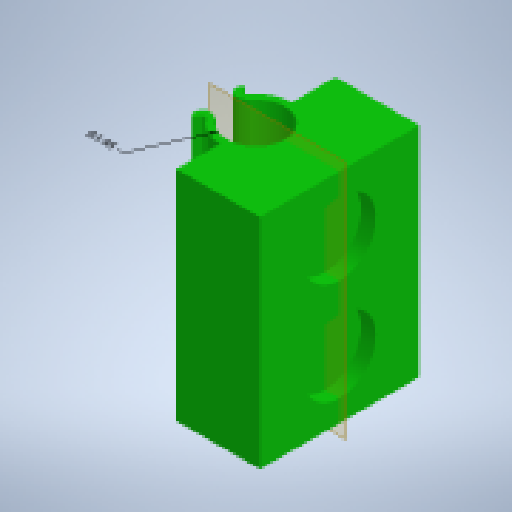
# Autodesk Inventor part: крепление маркера 8мм
Saved by Autodesk Inventor 2024.2 (Build 282272000, 272)
## iProperties
Created: 2025-12-12
Part Number: крепление маркера 8мм
Material: Типовые
Document SubType Name: Modeling
Designer: katya_notebook
Density: 1 g/cm^3
Appearance: Темно-зеленый
Author: katya_notebook
Autodesk Inventor part; units mm, degrees
ref_plane "YZ Plane" through (0, 0, 0) normal (1, 0, 0) x (0, 1, 0)
ref_plane "XZ Plane" through (0, 0, 0) normal (0, 1, 0) x (-1, 0, 0)
sketch "Эскиз1" plane through (0, 0, 0) normal (0, 1, 0) x (-1, 0, 0)
  circle A0 centre (0, 0) radius 3.95
  circle A1 centre (0, 0) radius 4.95
  line L0 (0, 0) -> (3.95, 2.9833)
  line L1 (0, 0) -> (3.95, -2.9833)
  point P0 (3.152, -2.3806)
  point P1 (3.152, 2.3806)
  dimension "d0" = 7.9
  dimension "d1" = 9.9
  constraints: 4 end point, 2 centre point, 2 coincident, 2 point on circle
  measures "d0" diameter of A0
  measures "d1" diameter of A1
extrude "Выдавливание1" add sketch "Эскиз1" along normal blind 30 contours A0 L1 A1 L0 picked at (3.1693, 3.3115)
sketch "Эскиз2" plane through (0, 30, 0) normal (0, 1, 0) x (1, 0, 0)
  arc A0 (-3.152, -2.3806) -> (-4.0447, -1.8507) centre (-5.8533, -5.9145) ccw
  arc A1 (-4.0447, -1.8507) -> (-5.2016, -3.6565) centre (-4.4791, -2.8459) ccw
  line L0 (-5.2016, -3.6565) -> (-4.5303, -2.802)
  arc A2 (-3.9514, -2.9687) -> (-4.5303, -2.802) centre (-4.3197, -3.1592) ccw
  line L1 (0, 0) -> (-3.2711, 0)
  arc A3 (-4.0447, 1.8507) -> (-3.152, 2.3806) centre (-5.8533, 5.9145) ccw
  arc A4 (-5.2016, 3.6565) -> (-4.0447, 1.8507) centre (-4.4791, 2.8459) ccw
  line L2 (-5.2016, 3.6565) -> (-4.5303, 2.802)
  arc A5 (-4.5303, 2.802) -> (-3.9514, 2.9687) centre (-4.3197, 3.1592) ccw
  line L3 (-3.152, -2.3806) -> (-3.95, -2.9833) projected
  line L4 (-3.95, -2.9833) -> (-3.152, -2.3806)
  line L5 (-3.95, -2.9833) -> (-3.9514, -2.9687)
  line L6 (-3.152, 2.3806) -> (-3.95, 2.9833)
  line L7 (-3.95, 2.9833) -> (-3.9514, 2.9687)
  constraints: 14 end point, 13 point on circle, 7 symmetric about line, 6 centre point, 1 coincident, 1 collinear, 1 horizontal, 3 other
extrude "Выдавливание2" add sketch "Эскиз2" against normal blind 30
sketch "Эскиз3" plane through (0, 30, 0) normal (0, 1, 0) x (1, 0, 0)
  arc A0 (-3.95, -2.9833) -> (-3.95, 2.9833) centre (0, 0) ccw projected
  line L0 (11.5, -6.95) -> (11.5, 6.95)
  arc A1 (-3.152, -2.3806) -> (-3.152, 2.3806) centre (0, 0) ccw projected
  arc A2 (0, -3.95) -> (0, 3.95) centre (0, 0) ccw
  line L1 (0, -4.95) -> (0, -3.95)
  line L2 (0, 3.95) -> (0, 4.95)
  line L3 (11.5, 6.95) -> (11.5, 10.95)
  line L4 (11.5, -6.95) -> (11.5, -10.95)
  line L5 (11.5, 10.95) -> (0, 10.95)
  line L6 (0, 10.95) -> (0, 4.95)
  line L7 (11.5, -10.95) -> (0, -10.95)
  line L8 (0, -10.95) -> (0, -4.95)
  dimension "d13" = 4
  dimension "d14" = 4
  dimension "d21" = 11.5
  dimension "d22" = 21.9
  dimension "d23" = 7
  constraints: 18 end point, 6 point on circle, 4 vertical, 2 horizontal, 2 perpendicular, 1 centre point, 1 collinear
  measures "d13" distance of L4.end L0.start
  measures "d14" distance of L3.end L0.end
  measures "d21" distance of L3.end L5.end
  measures "d22" distance of L4.end L3.end
  measures "d23" distance of L7.end L1.end
extrude "Выдавливание3" add sketch "Эскиз3" against normal blind 30 contours A0 L6 L5 L3 L0 L4 L7 L8
sketch "Эскиз5" plane through (11.5, 30, 10.95) normal (1, 0, 0) x (0, 0, -1)
  circle A0 centre (10.95, -22) radius 5 projected
  circle A1 centre (10.95, -22) radius 5
  circle A2 centre (10.95, -8) radius 5 projected
  circle A3 centre (10.95, -8) radius 5
  point P0 (10.95, -30)
  constraints: 2 centre point, 2 coincident
extrude "Выдавливание5" cut sketch "Эскиз5" against normal blind 2
